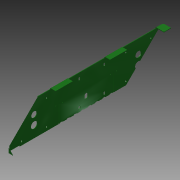
# Autodesk Inventor part: InnerSide
Saved by Autodesk Inventor 2014 (Build 180170000, 170)
## iProperties
Created: 2014-01-11
Part Number: InnerSide
Material: Generic
Document SubType Name: Sheet Metal
Designer: Alex
Density: 1 g/cm^3
Sheet Metal Rule: Default
Appearance: Smooth - Dark Forest Green
Mass: 262.954 g
Surface Area: 2370.16 cm^2
Volume: 262.954 cm^3
Author: Alex
Autodesk Inventor part; units mm, degrees
ref_plane "YZ Plane" through (0, 0, 0) normal (1, 0, 0) x (0, 1, 0)
ref_plane "XZ Plane" through (0, 0, 0) normal (0, 1, 0) x (-1, 0, 0)
ref_plane "XY Plane" through (0, 0, 0) normal (0, 0, 1) x (1, 0, 0)
sketch "Sketch1" plane through (0, 0, 0) normal (1, 0, 0) x (0, 1, 0)
  line L0 (196.2698, 454.4639) -> (43.8698, 454.4639)
  line L1 (43.8698, 454.4639) -> (43.8698, -237.9401)
  line L2 (43.8698, -237.9401) -> (196.2698, -237.9401)
  line L3 (196.2698, -237.9401) -> (196.2698, 454.4639)
  point P0 (0, 0)
  dimension "d0" = 152.4
  dimension "d1" = 692.404
  measures "d0" distance of L2.end L1.end
  measures "d1" distance of L1.end L0.end
extrude "Plate1" add sketch "Sketch1" along normal blind 2.286
sketch "Sketch2" plane through (0, 43.8698, 452.1779) normal (0, 0, 1) x (1, 0, 0)
  line L0 (0, 152.4) -> (0, 0)
  line L1 (0, 0) -> (25.4, 0)
  line L2 (25.4, 0) -> (25.4, 152.4)
  line L3 (25.4, 152.4) -> (0, 152.4)
  constraints: 6 end point, 1 horizontal, 1 perpendicular, 1 vertical
edge flange "Flange1" height 25.4 angle 90 thickness 2.286 bend radius 2.286 thickness toward (0, 0, 1) relief straight relief width 2.286 relief depth 1.143 corner gap 2.286 corner form 0 edges at (2.286, 120.0698, 454.4639) (2.286, 120.0698, -237.9401) wall of the first edge with corners at (0, 196.2698, 452.1779) (0, 43.8698, 452.1779) (25.4, 43.8698, 452.1779) (25.4, 196.2698, 452.1779)
bend "Bend1"
corner "Corner1"
sketch "Sketch3" plane through (0, 0, 0) normal (-1, 0, 0) x (0, 0, 1)
  line L0 (449.8919, 43.8698) -> (-233.3681, 43.8698) projected
  line L1 (-13.9121, 120.0698) -> (-13.9121, 196.2698) projected
  line L2 (-13.9121, 120.0698) -> (-11.6261, 120.0698) projected
  line L3 (-11.6261, 196.2698) -> (-11.6261, 120.0698) projected
  line L4 (-13.9121, 196.2698) -> (-11.6261, 196.2698) projected
  line L5 (228.1499, 120.0698) -> (228.1499, 196.2698) projected
  line L6 (228.1499, 120.0698) -> (230.4359, 120.0698) projected
  line L7 (230.4359, 196.2698) -> (230.4359, 120.0698) projected
  line L8 (228.1499, 196.2698) -> (230.4359, 196.2698) projected
  line L9 (-11.6261, 120.0698) -> (-13.9121, 120.0698)
  line L10 (-13.9121, 120.0698) -> (-13.9121, 43.8698)
  line L11 (-13.9121, 43.8698) -> (-11.6261, 43.8698)
  line L12 (-11.6261, 43.8698) -> (-11.6261, 120.0698)
  line L13 (230.4359, 120.0698) -> (228.1499, 120.0698)
  line L14 (228.1499, 120.0698) -> (228.1499, 43.8698)
  line L15 (228.1499, 43.8698) -> (230.4359, 43.8698)
  line L16 (230.4359, 43.8698) -> (230.4359, 120.0698)
  line L17 (-13.9121, 120.0698) -> (-11.6261, 120.0698)
  line L18 (-11.6261, 120.0698) -> (-11.6261, 43.8698)
  line L19 (-11.6261, 43.8698) -> (-13.9121, 43.8698)
  line L20 (-13.9121, 43.8698) -> (-13.9121, 120.0698)
  line L21 (228.1499, 120.0698) -> (230.4359, 120.0698)
  line L22 (230.4359, 120.0698) -> (230.4359, 43.8698)
  line L23 (230.4359, 43.8698) -> (228.1499, 43.8698)
  line L24 (228.1499, 43.8698) -> (228.1499, 120.0698)
  point P0 (0, 0)
  constraints: 32 end point, 8 parallel, 4 horizontal, 4 perpendicular, 2 point on line
extrude "Cut1" cut sketch "Sketch3" against normal blind 2.286 contours L0 L14 L6 L16 | L0 L10 L2 L12
sketch "Sketch4" plane through (2.286, 0, 0) normal (1, 0, 0) x (0, 0, -1)
  line L0 (233.3681, 43.8698) -> (233.3681, 196.2698)
  line L1 (-449.8919, 196.2698) -> (-449.8919, 43.8698)
  line L2 (-230.4359, 43.8698) -> (-230.4359, 120.0698)
  line L3 (11.6261, 43.8698) -> (-228.1499, 43.8698)
  circle A0 centre (-108.2619, 94.6698) radius 76.2 construction
  circle A1 centre (-340.1639, 94.6698) radius 76.2 construction
  circle A2 centre (123.6401, 94.6698) radius 76.2 construction
  circle A3 centre (-108.2619, 94.6698) radius 7.62
  circle A4 centre (-340.1639, 135.3606) radius 10.8585
  circle A5 centre (-340.1639, 94.6698) radius 14.2875
  circle A6 centre (123.6401, 135.3606) radius 10.8585
  circle A7 centre (123.6401, 94.6698) radius 14.2875
  line L4 (-402.8702, 178.5152) -> (-277.4577, 178.5152)
  arc A8 (-276.6639, 177.7214) -> (-277.4577, 178.5152) centre (-277.4577, 177.7214) ccw
  line L5 (-276.6639, 177.7214) -> (-276.6639, 52.3089)
  arc A9 (-277.4577, 51.5152) -> (-276.6639, 52.3089) centre (-277.4577, 52.3089) ccw
  line L6 (-277.4577, 51.5152) -> (-402.8702, 51.5152)
  arc A10 (-403.6639, 52.3089) -> (-402.8702, 51.5152) centre (-402.8702, 52.3089) ccw
  line L7 (-403.6639, 52.3089) -> (-403.6639, 177.7214)
  arc A11 (-402.8702, 178.5152) -> (-403.6639, 177.7214) centre (-402.8702, 177.7214) ccw
  circle A12 centre (-284.6014, 59.4527) radius 3.3528
  circle A13 centre (-340.1639, 135.3606) radius 11.1125
  circle A14 centre (-395.7264, 170.5777) radius 3.3528
  circle A15 centre (-378.3722, 146.7652) radius 5.5626
  circle A16 centre (-301.9557, 95.9652) radius 5.5626
  circle A17 centre (-301.9557, 121.3652) radius 5.5626
  circle A18 centre (-378.3722, 95.9652) radius 5.5626
  circle A19 centre (-301.9557, 146.7652) radius 5.5626
  circle A20 centre (-378.3722, 121.3652) radius 5.5626
  circle A21 centre (-340.1639, 94.6698) radius 14.2875
  circle A22 centre (-395.7264, 59.4527) radius 3.3528
  circle A23 centre (-284.6014, 170.5777) radius 3.3528
  line L8 (-146.3619, 57.3281) -> (-146.3619, 182.8041)
  arc A24 (-145.5999, 183.5661) -> (-146.3619, 182.8041) centre (-145.5999, 182.8041) ccw
  line L9 (-145.5999, 183.5661) -> (-20.1239, 183.5661)
  arc A25 (-19.3619, 182.8041) -> (-20.1239, 183.5661) centre (-20.1239, 182.8041) ccw
  line L10 (-19.3619, 182.8041) -> (-19.3619, 57.3281)
  arc A26 (-20.1239, 56.5661) -> (-19.3619, 57.3281) centre (-20.1239, 57.3281) ccw
  line L11 (-20.1239, 56.5661) -> (-145.5999, 56.5661)
  arc A27 (-146.3619, 57.3281) -> (-145.5999, 56.5661) centre (-145.5999, 57.3281) ccw
  circle A28 centre (-76.5119, 150.5461) radius 11.1062
  circle A29 centre (-52.1284, 174.4142) radius 4.3561
  circle A30 centre (-98.0514, 173.1776) radius 4.3561
  circle A31 centre (-108.2619, 94.6698) radius 14.2812
  circle A32 centre (-138.4371, 64.4909) radius 3.3528
  circle A33 centre (-27.2867, 175.6413) radius 3.3528
  circle A34 centre (-27.2867, 64.4909) radius 3.3528
  circle A35 centre (-138.4371, 175.6413) radius 3.3528
  circle A36 centre (-70.2635, 110.9806) radius 14.2812
  circle A37 centre (-34.7538, 126.6779) radius 4.3561
  circle A38 centre (-121.1141, 127.9145) radius 4.3561
  line L12 (60.9338, 178.5152) -> (186.3463, 178.5152)
  arc A39 (187.1401, 177.7214) -> (186.3463, 178.5152) centre (186.3463, 177.7214) ccw
  line L13 (187.1401, 177.7214) -> (187.1401, 52.3089)
  arc A40 (186.3463, 51.5152) -> (187.1401, 52.3089) centre (186.3463, 52.3089) ccw
  line L14 (186.3463, 51.5152) -> (60.9338, 51.5152)
  arc A41 (60.1401, 52.3089) -> (60.9338, 51.5152) centre (60.9338, 52.3089) ccw
  line L15 (60.1401, 52.3089) -> (60.1401, 177.7214)
  arc A42 (60.9338, 178.5152) -> (60.1401, 177.7214) centre (60.9338, 177.7214) ccw
  circle A43 centre (179.2026, 59.4527) radius 3.3528
  circle A44 centre (123.6401, 135.3606) radius 11.1125
  circle A45 centre (68.0776, 170.5777) radius 3.3528
  circle A46 centre (85.4318, 146.7652) radius 5.5626
  circle A47 centre (161.8483, 95.9652) radius 5.5626
  circle A48 centre (161.8483, 121.3652) radius 5.5626
  circle A49 centre (85.4318, 95.9652) radius 5.5626
  circle A50 centre (161.8483, 146.7652) radius 5.5626
  circle A51 centre (85.4318, 121.3652) radius 5.5626
  circle A52 centre (123.6401, 94.6698) radius 14.2875
  circle A53 centre (68.0776, 59.4527) radius 3.3528
  circle A54 centre (179.2026, 170.5777) radius 3.3528
  circle A55 centre (-340.1639, 94.6698) radius 14.2875
  circle A56 centre (-340.1639, 135.3606) radius 10.8585
  circle A57 centre (-395.7264, 170.5777) radius 3.3528
  circle A58 centre (-284.6014, 170.5777) radius 3.3528
  circle A59 centre (-284.6014, 59.4527) radius 3.3528
  circle A60 centre (-395.7264, 59.4527) radius 3.3528
  circle A61 centre (-138.4371, 64.4909) radius 3.3528
  circle A62 centre (-138.4371, 175.6413) radius 3.3528
  circle A63 centre (-27.2867, 175.6413) radius 3.3528
  circle A64 centre (-27.2867, 64.4909) radius 3.3528
  circle A65 centre (68.0776, 59.4527) radius 3.3528
  circle A66 centre (123.6401, 94.6698) radius 14.2875
  circle A67 centre (123.6401, 135.3606) radius 11.1125
  circle A68 centre (68.0776, 170.5777) radius 3.3528
  circle A69 centre (179.2026, 170.5777) radius 3.3528
  circle A70 centre (179.2026, 59.4527) radius 3.3528
  line L16 (-108.2619, 94.6698) -> (-108.2619, 88.3198) construction
  line L17 (-115.8819, 94.6698) -> (-115.8819, 88.3198)
  line L18 (-100.6419, 88.3198) -> (-100.6419, 94.6698)
  arc A71 (-100.6419, 94.6698) -> (-115.8819, 94.6698) centre (-108.2619, 94.6698) ccw
  arc A72 (-115.8819, 88.3198) -> (-100.6419, 88.3198) centre (-108.2619, 88.3198) ccw
  line L19 (-138.4371, 64.4909) -> (-138.4371, 58.1409) construction
  line L20 (-141.7899, 64.4909) -> (-141.7899, 58.1409)
  line L21 (-135.0843, 58.1409) -> (-135.0843, 64.4909)
  arc A73 (-135.0843, 64.4909) -> (-141.7899, 64.4909) centre (-138.4371, 64.4909) ccw
  arc A74 (-141.7899, 58.1409) -> (-135.0843, 58.1409) centre (-138.4371, 58.1409) ccw
  line L22 (-138.4371, 175.6413) -> (-138.4371, 169.2913) construction
  line L23 (-141.7899, 175.6413) -> (-141.7899, 169.2913)
  line L24 (-135.0843, 169.2913) -> (-135.0843, 175.6413)
  arc A75 (-135.0843, 175.6413) -> (-141.7899, 175.6413) centre (-138.4371, 175.6413) ccw
  arc A76 (-141.7899, 169.2913) -> (-135.0843, 169.2913) centre (-138.4371, 169.2913) ccw
  line L25 (-27.2867, 175.6413) -> (-27.2867, 169.2913) construction
  line L26 (-30.6395, 175.6413) -> (-30.6395, 169.2913)
  line L27 (-23.9339, 169.2913) -> (-23.9339, 175.6413)
  arc A77 (-23.9339, 175.6413) -> (-30.6395, 175.6413) centre (-27.2867, 175.6413) ccw
  arc A78 (-30.6395, 169.2913) -> (-23.9339, 169.2913) centre (-27.2867, 169.2913) ccw
  line L28 (-27.2867, 64.4909) -> (-27.2867, 58.1409) construction
  line L29 (-30.6395, 64.4909) -> (-30.6395, 58.1409)
  line L30 (-23.9339, 58.1409) -> (-23.9339, 64.4909)
  arc A79 (-23.9339, 64.4909) -> (-30.6395, 64.4909) centre (-27.2867, 64.4909) ccw
  arc A80 (-30.6395, 58.1409) -> (-23.9339, 58.1409) centre (-27.2867, 58.1409) ccw
  circle A81 centre (-340.1639, 135.3606) radius 12.7
  circle A82 centre (123.6401, 135.3606) radius 12.7
  point P0 (0, 0)
  point P1 (-108.2619, 91.4948)
  point P2 (-138.4371, 61.3159)
  point P3 (-138.4371, 172.4663)
  point P4 (-27.2867, 172.4663)
  point P5 (-27.2867, 61.3159)
extrude "Cut2" cut sketch "Sketch4" against normal blind 2.286 contours A3 | L18 A72 L17 A3 | A4 | A5 | A6 | A7 | A12 | A13 | A14 | A22 | A23 | A74 L20 A32 L21 L11 | L11 A74 | A80 L29 A34 L30 L11 | L11 A80 | A32 | A34 | A33 | L27 A78 L26 A33 | A35 | L24 A76 L23 A35 | A43 | A44 | A45 | A53 | A54 | A81 | A82
sketch "Sketch7" plane through (0, 0, 0) normal (-1, 0, 0) x (0, 0, 1)
  line L0 (-233.3681, 196.2698) -> (449.8919, 196.2698)
  line L1 (-233.3681, 196.2698) -> (-202.1261, 196.2698)
  line L2 (-202.1261, 196.2698) -> (-202.1261, 198.5558)
  line L3 (-202.1261, 198.5558) -> (-233.3681, 198.5558)
  line L4 (-233.3681, 198.5558) -> (-233.3681, 196.2698)
  line L5 (449.8919, 196.2698) -> (418.6499, 196.2698)
  line L6 (418.6499, 196.2698) -> (418.6499, 198.5558)
  line L7 (418.6499, 198.5558) -> (449.8919, 198.5558)
  line L8 (449.8919, 198.5558) -> (449.8919, 196.2698)
  point P0 (-52.0121, 196.2698)
  point P1 (0, 0)
  dimension "d50" = 31.242
  dimension "d51" = 2.286
  dimension "d52" = 31.242
  dimension "d53" = 2.286
  measures "d50" distance of L3.end L2.end
  measures "d51" distance between parallel lines of L3 L0
  measures "d52" distance of L6.end L7.end
  measures "d53" distance between parallel lines of L5 L7
sheet face with bend "Face2" sketch "Sketch7" thickness 2.286 toward (1, 0, 0) bend radius 2.286 relief straight relief width 2.286 relief depth 1.143
bend "Bend3"
sketch "Sketch8" plane through (2.286, 198.5558, -202.1261) normal (0, 1, 0) x (-1, 0, 0)
  line L0 (0, -31.242) -> (0, 0)
  line L1 (0, 0) -> (-35.814, 0)
  line L2 (-35.814, 0) -> (-35.814, -31.242)
  line L3 (-35.814, -31.242) -> (0, -31.242)
  constraints: 6 end point, 1 horizontal, 1 perpendicular, 1 vertical
edge flange "Flange3" height 38.1 angle 90 thickness 2.286 bend radius 2.286 thickness toward (0, 1, 0) relief straight relief width 2.286 relief depth 1.143 corner gap 2.286 corner form 0 edges at (2.286, 198.5558, -217.7471) (2.286, 198.5558, 434.2709) wall of the first edge with corners at (2.286, 198.5558, -233.3681) (2.286, 198.5558, -202.1261) (38.1, 198.5558, -202.1261) (38.1, 198.5558, -233.3681)
bend "Bend4"
corner "Corner3"
sketch "Sketch9" plane through (0, 0, 0) normal (-1, 0, 0) x (0, 0, 1)
  line L0 (-50.8691, 196.2698) -> (25.3309, 196.2698)
  line L1 (25.3309, 196.2698) -> (25.3309, 198.5558)
  line L2 (25.3309, 198.5558) -> (-50.8691, 198.5558)
  line L3 (-50.8691, 198.5558) -> (-50.8691, 196.2698)
  line L4 (191.1929, 196.2698) -> (267.3929, 196.2698)
  line L5 (267.3929, 196.2698) -> (267.3929, 198.5558)
  line L6 (267.3929, 198.5558) -> (191.1929, 198.5558)
  line L7 (191.1929, 198.5558) -> (191.1929, 196.2698)
  point P0 (0, 0)
  point P1 (267.3929, 196.2698)
  point P2 (25.3309, 196.2698)
  dimension "d69" = 2.286
  dimension "d70" = 2.286
  measures "d69" distance of L1.end L0.end
  measures "d70" distance of L5.end L4.end
sheet face with bend "Face3" sketch "Sketch9" thickness 2.286 toward (1, 0, 0) bend radius 2.286 relief straight relief width 2.286 relief depth 1.143
bend "Bend5"
sketch "Sketch10" plane through (2.286, 198.5558, 25.3309) normal (0, 1, 0) x (-1, 0, 0)
  line L0 (0, -76.2) -> (0, 0)
  line L1 (0, 0) -> (-23.114, 0)
  line L2 (-23.114, 0) -> (-23.114, -76.2)
  line L3 (-23.114, -76.2) -> (0, -76.2)
  constraints: 6 end point, 1 horizontal, 1 perpendicular, 1 vertical
edge flange "Flange4" height 25.4 angle 90 thickness 2.286 bend radius 2.286 thickness toward (0, 1, 0) relief straight relief width 2.286 relief depth 1.143 corner gap 2.286 corner form 0 edges at (2.286, 198.5558, -12.7691) (2.286, 198.5558, 229.2929) wall of the first edge with corners at (2.286, 198.5558, -50.8691) (2.286, 198.5558, 25.3309) (25.4, 198.5558, 25.3309) (25.4, 198.5558, -50.8691)
bend "Bend6"
corner "Corner4"
sketch "Sketch11" plane through (2.286, 0, 0) normal (1, 0, 0) x (0, 0, -1)
  line L0 (11.6261, 43.8698) -> (-228.1499, 43.8698) projected
  line L1 (-162.1099, 44.1238) -> (-149.4099, 44.1238) projected
  line L2 (-149.4099, 46.4098) -> (-149.4099, 44.1238) projected
  line L3 (-162.1099, 46.4098) -> (-149.4099, 46.4098) projected
  line L4 (-162.1099, 46.4098) -> (-162.1099, 44.1238) projected
  line L5 (-130.3599, 44.1238) -> (-117.6599, 44.1238) projected
  line L6 (-117.6599, 46.4098) -> (-117.6599, 44.1238) projected
  line L7 (-130.3599, 46.4098) -> (-117.6599, 46.4098) projected
  line L8 (-130.3599, 46.4098) -> (-130.3599, 44.1238) projected
  line L9 (-98.6099, 44.1238) -> (-86.1639, 44.1238) projected
  line L10 (-86.1639, 46.4098) -> (-86.1639, 44.1238) projected
  line L11 (-98.6099, 46.4098) -> (-86.1639, 46.4098) projected
  line L12 (-98.6099, 46.4098) -> (-98.6099, 44.1238) projected
  line L13 (-67.1139, 44.1238) -> (-54.4139, 44.1238) projected
  line L14 (-54.4139, 46.4098) -> (-54.4139, 44.1238) projected
  line L15 (-67.1139, 46.4098) -> (-54.4139, 46.4098) projected
  line L16 (-67.1139, 46.4098) -> (-67.1139, 44.1238) projected
  line L17 (-35.3639, 44.1238) -> (-22.6639, 44.1238) projected
  line L18 (-22.6639, 46.4098) -> (-22.6639, 44.1238) projected
  line L19 (-35.3639, 46.4098) -> (-22.6639, 46.4098) projected
  line L20 (-35.3639, 46.4098) -> (-35.3639, 44.1238) projected
  line L21 (-3.6139, 44.1238) -> (9.0861, 44.1238) projected
  line L22 (9.0861, 46.4098) -> (9.0861, 44.1238) projected
  line L23 (-3.6139, 46.4098) -> (9.0861, 46.4098) projected
  line L24 (-3.6139, 46.4098) -> (-3.6139, 44.1238) projected
  line L25 (-193.8599, 44.1238) -> (-181.1599, 44.1238) projected
  line L26 (-181.1599, 46.4098) -> (-181.1599, 44.1238) projected
  line L27 (-193.8599, 46.4098) -> (-181.1599, 46.4098) projected
  line L28 (-193.8599, 46.4098) -> (-193.8599, 44.1238) projected
  line L29 (-225.6099, 44.1238) -> (-212.9099, 44.1238) projected
  line L30 (-212.9099, 46.4098) -> (-212.9099, 44.1238) projected
  line L31 (-225.6099, 46.4098) -> (-212.9099, 46.4098) projected
  line L32 (-225.6099, 46.4098) -> (-225.6099, 44.1238) projected
  line L33 (-225.6099, 43.8698) -> (-212.9099, 43.8698)
  line L34 (-212.9099, 43.8698) -> (-212.9099, 46.4098)
  line L35 (-212.9099, 46.4098) -> (-225.6099, 46.4098)
  line L36 (-225.6099, 46.4098) -> (-225.6099, 43.8698)
  line L37 (-193.8599, 43.8698) -> (-181.1599, 43.8698)
  line L38 (-181.1599, 43.8698) -> (-181.1599, 46.4098)
  line L39 (-181.1599, 46.4098) -> (-193.8599, 46.4098)
  line L40 (-193.8599, 46.4098) -> (-193.8599, 43.8698)
  line L41 (-149.4099, 43.8698) -> (-162.1099, 43.8698)
  line L42 (-162.1099, 43.8698) -> (-162.1099, 46.4098)
  line L43 (-162.1099, 46.4098) -> (-149.4099, 46.4098)
  line L44 (-149.4099, 46.4098) -> (-149.4099, 43.8698)
  line L45 (-117.6599, 43.8698) -> (-130.3599, 43.8698)
  line L46 (-130.3599, 43.8698) -> (-130.3599, 46.4098)
  line L47 (-130.3599, 46.4098) -> (-117.6599, 46.4098)
  line L48 (-117.6599, 46.4098) -> (-117.6599, 43.8698)
  line L49 (-86.1639, 43.8698) -> (-98.6099, 43.8698)
  line L50 (-98.6099, 43.8698) -> (-98.6099, 46.4098)
  line L51 (-98.6099, 46.4098) -> (-86.1639, 46.4098)
  line L52 (-86.1639, 46.4098) -> (-86.1639, 43.8698)
  line L53 (-54.4139, 43.8698) -> (-67.1139, 43.8698)
  line L54 (-67.1139, 43.8698) -> (-67.1139, 46.4098)
  line L55 (-67.1139, 46.4098) -> (-54.4139, 46.4098)
  line L56 (-54.4139, 46.4098) -> (-54.4139, 43.8698)
  line L57 (-22.6639, 43.8698) -> (-35.3639, 43.8698)
  line L58 (-35.3639, 43.8698) -> (-35.3639, 46.4098)
  line L59 (-35.3639, 46.4098) -> (-22.6639, 46.4098)
  line L60 (-22.6639, 46.4098) -> (-22.6639, 43.8698)
  line L61 (9.0861, 43.8698) -> (-3.6139, 43.8698)
  line L62 (-3.6139, 43.8698) -> (-3.6139, 46.4098)
  line L63 (-3.6139, 46.4098) -> (9.0861, 46.4098)
  line L64 (9.0861, 46.4098) -> (9.0861, 43.8698)
  point P0 (0, 0)
  constraints: 64 end point, 16 parallel, 8 horizontal, 8 perpendicular, 9 other
extrude "Cut4" cut sketch "Sketch11" against normal blind 2.286
sketch "Sketch12" plane through (25.4, 43.8698, 454.4639) normal (0, 0, 1) x (1, 0, 0)
  line L0 (-25.4, 0) -> (-25.4, 152.4) projected
  line L1 (-20.828, 152.4) -> (-25.4, 152.4) projected
  line L2 (0, 152.4) -> (-25.4, 152.4)
  line L3 (-25.4, 152.4) -> (-25.4, 76.2)
  line L4 (-25.4, 76.2) -> (0, 76.2)
  line L5 (0, 76.2) -> (0, 152.4)
  point P0 (-25.4, -43.8698)
  dimension "d88" = 76.2
  constraints: 8 end point, 2 parallel, 1 horizontal, 1 midpoint, 1 perpendicular
  measures "d88" distance of L3.end L2.end
extrude "Cut5" cut sketch "Sketch12" against normal blind 4.572
sketch "Sketch13" plane through (25.4, 43.8698, -237.9401) normal (0, 0, -1) x (-1, 0, 0)
  line L0 (25.4, 152.4) -> (25.4, 0) projected
  line L1 (0, 152.4) -> (25.4, 152.4)
  line L2 (25.4, 152.4) -> (25.4, 76.2)
  line L3 (25.4, 76.2) -> (0, 76.2)
  line L4 (0, 76.2) -> (0, 152.4)
  point P0 (25.4, -43.8698)
  dimension "d91" = 76.2
  constraints: 8 end point, 2 parallel, 1 horizontal, 1 midpoint, 1 perpendicular
  measures "d91" distance of L1.end L2.end
extrude "Cut6" cut sketch "Sketch13" against normal blind 4.572
sketch "Sketch14" plane through (25.4, 43.8698, -237.9401) normal (0, 0, -1) x (-1, 0, 0)
  circle A0 centre (10.414, 50.8) radius 1.5875
  point P0 (25.4, -43.8698)
  constraints: 1 centre point, 2 other
extrude "Cut7" cut sketch "Sketch14" against normal through all
sketch "Sketch15" plane through (0, 0, 0) normal (-1, 0, 0) x (0, 0, 1)
  line L0 (449.8919, 43.8698) -> (230.4359, 43.8698) projected
  line L1 (-13.9121, 43.8698) -> (-233.3681, 43.8698) projected
  line L2 (449.8919, 48.4418) -> (403.6639, 48.4418)
  line L3 (-233.3681, 48.4418) -> (-187.1401, 48.4418)
  line L4 (-233.3681, 48.4418) -> (-187.0131, 48.4418)
  line L5 (-187.0131, 48.4418) -> (-187.0131, 43.8698)
  line L6 (-187.0131, 43.8698) -> (-233.3681, 43.8698)
  line L7 (-233.3681, 43.8698) -> (-233.3681, 48.4418)
  line L8 (449.8919, 48.4418) -> (403.5369, 48.4418)
  line L9 (403.5369, 48.4418) -> (403.5369, 43.8698)
  line L10 (403.5369, 43.8698) -> (449.8919, 43.8698)
  line L11 (449.8919, 43.8698) -> (449.8919, 48.4418)
  line L12 (449.8919, 48.4418) -> (403.6639, 48.4418)
  line L13 (449.8919, 48.4418) -> (403.6639, 48.4418)
  line L14 (-187.1401, 48.4418) -> (-233.3681, 48.4418)
  line L15 (-187.1401, 48.4418) -> (-233.3681, 48.4418)
  line L16 (-187.1401, 48.4418) -> (-233.3681, 48.4418)
  line L17 (-187.1401, 48.4418) -> (-233.3681, 48.4418)
  line L18 (-187.1401, 48.4418) -> (-233.3681, 48.4418)
  line L19 (-187.1401, 48.4418) -> (-233.3681, 48.4418)
  line L20 (-187.1401, 48.4418) -> (-233.3681, 48.4418)
  line L21 (35.3639, 46.4098) -> (35.3639, 43.8698) projected
  line L22 (54.4139, 43.8698) -> (35.3639, 43.8698) projected
  line L23 (54.4139, 43.8698) -> (54.4139, 46.4098) projected
  line L24 (54.4139, 46.4098) -> (67.1139, 46.4098) projected
  line L25 (67.1139, 46.4098) -> (67.1139, 43.8698) projected
  line L26 (86.1639, 43.8698) -> (67.1139, 43.8698) projected
  line L27 (86.1639, 43.8698) -> (86.1639, 46.4098) projected
  line L28 (86.1639, 46.4098) -> (98.6099, 46.4098) projected
  line L29 (98.6099, 46.4098) -> (98.6099, 43.8698) projected
  line L30 (117.6599, 43.8698) -> (98.6099, 43.8698) projected
  line L31 (117.6599, 43.8698) -> (117.6599, 46.4098) projected
  line L32 (117.6599, 46.4098) -> (130.3599, 46.4098) projected
  line L33 (130.3599, 46.4098) -> (130.3599, 43.8698) projected
  line L34 (149.4099, 43.8698) -> (130.3599, 43.8698) projected
  line L35 (149.4099, 43.8698) -> (149.4099, 46.4098) projected
  line L36 (149.4099, 46.4098) -> (162.1099, 46.4098) projected
  line L37 (162.1099, 46.4098) -> (162.1099, 43.8698) projected
  line L38 (181.1599, 43.8698) -> (162.1099, 43.8698) projected
  line L39 (181.1599, 43.8698) -> (181.1599, 46.4098) projected
  line L40 (181.1599, 46.4098) -> (193.8599, 46.4098) projected
  line L41 (193.8599, 46.4098) -> (193.8599, 43.8698) projected
  line L42 (212.9099, 43.8698) -> (193.8599, 43.8698) projected
  line L43 (212.9099, 43.8698) -> (212.9099, 46.4098) projected
  line L44 (212.9099, 46.4098) -> (225.6099, 46.4098) projected
  line L45 (225.6099, 46.4098) -> (225.6099, 43.8698) projected
  line L46 (228.1499, 43.8698) -> (225.6099, 43.8698) projected
  line L47 (228.1499, 43.8698) -> (228.1499, 120.0698) projected
  line L48 (228.1499, 120.0698) -> (230.4359, 120.0698) projected
  line L49 (230.4359, 120.0698) -> (230.4359, 43.8698) projected
  line L50 (449.8919, 43.8698) -> (230.4359, 43.8698) projected
  line L51 (449.8919, 43.8698) -> (449.8919, 120.0698) projected
  line L52 (449.8919, 120.0698) -> (449.8919, 196.2698) projected
  line L53 (418.6499, 196.2698) -> (449.8919, 196.2698) projected
  line L54 (267.3929, 196.2698) -> (418.6499, 196.2698) projected
  line L55 (191.1929, 196.2698) -> (267.3929, 196.2698) projected
  line L56 (25.3309, 196.2698) -> (191.1929, 196.2698) projected
  line L57 (-50.8691, 196.2698) -> (25.3309, 196.2698) projected
  line L58 (-202.1261, 196.2698) -> (-50.8691, 196.2698) projected
  line L59 (-233.3681, 196.2698) -> (-202.1261, 196.2698) projected
  line L60 (-233.3681, 196.2698) -> (-233.3681, 120.0698) projected
  line L61 (-233.3681, 120.0698) -> (-233.3681, 43.8698) projected
  line L62 (-13.9121, 43.8698) -> (-233.3681, 43.8698) projected
  line L63 (-13.9121, 43.8698) -> (-13.9121, 120.0698) projected
  line L64 (-13.9121, 120.0698) -> (-11.6261, 120.0698) projected
  line L65 (-11.6261, 120.0698) -> (-11.6261, 43.8698) projected
  line L66 (-9.0861, 43.8698) -> (-11.6261, 43.8698) projected
  line L67 (-9.0861, 43.8698) -> (-9.0861, 46.4098) projected
  line L68 (-9.0861, 46.4098) -> (3.6139, 46.4098) projected
  line L69 (3.6139, 46.4098) -> (3.6139, 43.8698) projected
  line L70 (22.6639, 43.8698) -> (3.6139, 43.8698) projected
  line L71 (22.6639, 43.8698) -> (22.6639, 46.4098) projected
  line L72 (22.6639, 46.4098) -> (35.3639, 46.4098) projected
  arc A0 (100.6419, 88.3198) -> (115.8819, 88.3198) centre (108.2619, 88.3198) ccw projected
  line L73 (100.6419, 88.3198) -> (100.6419, 94.6698) projected
  arc A1 (115.8819, 94.6698) -> (100.6419, 94.6698) centre (108.2619, 94.6698) ccw projected
  line L74 (115.8819, 94.6698) -> (115.8819, 88.3198) projected
  arc A2 (23.9339, 169.2913) -> (30.6395, 169.2913) centre (27.2867, 169.2913) ccw projected
  line L75 (23.9339, 169.2913) -> (23.9339, 175.6413) projected
  arc A3 (30.6395, 175.6413) -> (23.9339, 175.6413) centre (27.2867, 175.6413) ccw projected
  line L76 (30.6395, 175.6413) -> (30.6395, 169.2913) projected
  circle A4 centre (-123.6401, 135.3606) radius 12.7 projected
  circle A5 centre (-68.0776, 59.4527) radius 3.3528 projected
  circle A6 centre (-179.2026, 59.4527) radius 3.3528 projected
  circle A7 centre (340.1639, 135.3606) radius 12.7 projected
  circle A8 centre (395.7264, 59.4527) radius 3.3528 projected
  circle A9 centre (284.6014, 59.4527) radius 3.3528 projected
  arc A10 (135.0843, 58.1409) -> (141.7899, 58.1409) centre (138.4371, 58.1409) ccw projected
  line L77 (135.0843, 58.1409) -> (135.0843, 64.4909) projected
  arc A11 (141.7899, 64.4909) -> (135.0843, 64.4909) centre (138.4371, 64.4909) ccw projected
  line L78 (141.7899, 64.4909) -> (141.7899, 58.1409) projected
  arc A12 (23.9339, 58.1409) -> (30.6395, 58.1409) centre (27.2867, 58.1409) ccw projected
  line L79 (23.9339, 58.1409) -> (23.9339, 64.4909) projected
  arc A13 (30.6395, 64.4909) -> (23.9339, 64.4909) centre (27.2867, 64.4909) ccw projected
  line L80 (30.6395, 64.4909) -> (30.6395, 58.1409) projected
  circle A14 centre (395.7264, 170.5777) radius 3.3528 projected
  circle A15 centre (284.6014, 170.5777) radius 3.3528 projected
  circle A16 centre (340.1639, 94.6698) radius 14.2875 projected
  circle A17 centre (-68.0776, 170.5777) radius 3.3528 projected
  circle A18 centre (-179.2026, 170.5777) radius 3.3528 projected
  circle A19 centre (-123.6401, 94.6698) radius 14.2875 projected
  arc A20 (135.0843, 169.2913) -> (141.7899, 169.2913) centre (138.4371, 169.2913) ccw projected
  line L81 (135.0843, 169.2913) -> (135.0843, 175.6413) projected
  arc A21 (141.7899, 175.6413) -> (135.0843, 175.6413) centre (138.4371, 175.6413) ccw projected
  line L82 (141.7899, 175.6413) -> (141.7899, 169.2913) projected
  line L83 (-187.1401, 48.4418) -> (-233.3681, 48.4418)
  line L84 (-187.1401, 48.4418) -> (-233.3681, 48.4418)
  line L85 (-233.3681, 48.4418) -> (-187.1401, 48.4418)
  line L86 (-233.3681, 48.4418) -> (-187.1401, 48.4418)
  line L87 (-233.3681, 48.4418) -> (-187.1401, 48.4418)
  line L88 (-187.0131, 43.8698) -> (-241.061, 43.8698)
  line L89 (-241.061, 43.8698) -> (-241.061, 48.4418)
  line L90 (-241.061, 48.4418) -> (-187.0131, 48.4418)
  line L91 (-187.0131, 48.4418) -> (-187.0131, 43.8698)
  line L92 (403.5369, 43.8698) -> (457.1836, 43.8698)
  line L93 (457.1836, 43.8698) -> (457.1836, 48.4418)
  line L94 (457.1836, 48.4418) -> (403.5369, 48.4418)
  line L95 (403.5369, 48.4418) -> (403.5369, 43.8698)
  point P0 (0, 0)
  dimension "d96" = 46.355
  dimension "d97" = 46.355
  constraints: 64 end point, 20 horizontal, 8 parallel, 4 perpendicular, 4 point on line, 4 other
  measures "d96" distance of L3.start L4.end
  measures "d97" distance of L10.end L9.end
extrude "Cut8" cut sketch "Sketch15" against normal blind 2.286 contours L0 L9 L8 L2 L11 | L3 L4 L5 L1 L7
sketch "Sketch16" plane through (0, 0, 0) normal (-1, 0, 0) x (0, 0, 1)
  circle A0 centre (-26.8661, 120.0698) radius 1.5878
  circle A1 centre (1.3279, 120.0698) radius 1.5875
  circle A2 centre (-26.8661, 120.0698) radius 1.5878
  circle A3 centre (215.1959, 120.0698) radius 1.5875
  circle A4 centre (243.3899, 120.0698) radius 1.5875
  line L0 (-50.8691, 196.2698) -> (25.3309, 196.2698) projected
  circle A5 centre (-26.8661, 183.5698) radius 1.5875
  circle A6 centre (1.3279, 183.5698) radius 1.5875
  circle A7 centre (215.1959, 185.1573) radius 1.5875
  circle A8 centre (243.3899, 185.1573) radius 1.5875
  point P0 (0, 0)
  dimension "d102" = 3.175
  dimension "d103" = 12.7
  constraints: 9 centre point, 10 other
  measures "d102" diameter of A5
  measures "d103" distance from line of L0 A5.centre
extrude "Cut9" cut sketch "Sketch16" against normal blind 2.286 contours A5 | A6 | A7 | A8
equation "\"d13\" = Thickness"
equation "\"d22\" = Thickness"
equation "\"d86\" = Thickness"
equation "\"d94\" = Thickness"
equation "\"d98\" = Thickness"
equation "\"d100\" = Thickness"
equation "\"d3\" = BendReliefWidth"
equation "\"d4\" = BendReliefDepth"
equation "\"d5\" = MinimumRemnant"
equation "\"d6\" = BendRadius"
equation "\"d9\" = BendRadius"
equation "\"d10\" = CornerReliefSize"
equation "\"d11\" = GapSize"
equation "\"d12\" = JacobiRadiusSize"
equation "\"d54\" = BendRadius"
equation "\"d55\" = BendReliefWidth"
equation "\"d57\" = MinimumRemnant"
equation "\"d56\" = BendReliefDepth"
equation "\"d58\" = BendRadius"
equation "\"d59\" = BendReliefWidth"
equation "\"d60\" = BendReliefDepth"
equation "\"d61\" = MinimumRemnant"
equation "\"d62\" = BendRadius"
equation "\"d65\" = BendRadius"
equation "\"d66\" = CornerReliefSize"
equation "\"d67\" = GapSize"
equation "\"d68\" = JacobiRadiusSize"
equation "\"d71\" = BendRadius"
equation "\"d72\" = BendReliefWidth"
equation "\"d74\" = MinimumRemnant"
equation "\"d73\" = BendReliefDepth"
equation "\"d75\" = BendRadius"
equation "\"d76\" = BendReliefWidth"
equation "\"d77\" = BendReliefDepth"
equation "\"d78\" = MinimumRemnant"
equation "\"d79\" = BendRadius"
equation "\"d82\" = BendRadius"
equation "\"d83\" = CornerReliefSize"
equation "\"d84\" = GapSize"
equation "\"d85\" = JacobiRadiusSize"
equation "\"BendRadius\" = Thickness"
equation "\"BendReliefWidth\" = Thickness"
equation "\"BendReliefDepth\" = 0.5 * Thickness"
equation "\"CornerReliefSize\" = 4 * Thickness"
equation "\"MinimumRemnant\" = 2 * Thickness"
equation "\"TransitionRadius\" = BendRadius"
equation "\"JacobiRadiusSize\" = BendRadius"
equation "\"GapSize\" = Thickness"
equation "\"d2\" = BendRadius"
equation "\"d17\" = d18"
equation "\"d19\" = d20"
equation "\"Thickness\" = 2.286"
equation "\"d18\" = 341.63"
equation "\"d20\" = 109.728"
body "Solid1"
